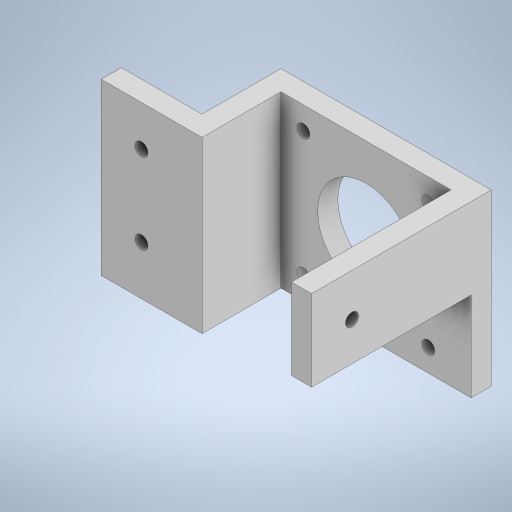
# Autodesk Inventor part: Motor Mount
Saved by Autodesk Inventor 2023.1 (Build 271208000, 208)
## iProperties
Created: 2022-10-30
Part Number: Motor Mount
Material: Generic
Document SubType Name: Modeling
Designer: nicol
Density: 1 g/cm^3
Appearance: Default
Author: nicol
Autodesk Inventor part; units mm, degrees
ref_plane "YZ Plane" through (0, 0, 0) normal (1, 0, 0) x (0, 1, 0)
ref_plane "XZ Plane" through (0, 0, 0) normal (0, 1, 0) x (-1, 0, 0)
ref_plane "XY Plane" through (0, 0, 0) normal (0, 0, 1) x (1, 0, 0)
sketch "Sketch1" plane through (0, 0, 0) normal (0, 0, 1) x (1, 0, 0)
  line L0 (0, 0) -> (42.2, 0)
  line L1 (42.2, 0) -> (42.2, 42.2)
  line L2 (42.2, 42.2) -> (0, 42.2)
  line L3 (0, 42.2) -> (0, 0)
  line L4 (0, 0) -> (5, 0)
  line L5 (42.2, 0) -> (45, 0)
  line L6 (5.6, 36.6) -> (36.6, 36.6) construction
  line L7 (36.6, 36.6) -> (36.6, 5.6) construction
  line L8 (36.6, 5.6) -> (5.6, 5.6) construction
  line L9 (5.6, 5.6) -> (5.6, 36.6) construction
  circle A0 centre (21.1, 21.1) radius 12
  line L10 (0.1, 42.1) -> (42.1, 42.1)
  line L11 (42.1, 42.1) -> (42.1, 0.1)
  line L12 (42.1, 0.1) -> (0.1, 0.1)
  line L13 (0.1, 0.1) -> (0.1, 42.1)
  line L14 (42.2, 42.2) -> (47.2, 42.2)
  line L15 (47.2, 42.2) -> (47.2, 21.1)
  line L16 (47.2, 21.1) -> (42.2, 21.1)
  line L17 (42.2, 21.1) -> (42.2, 42.2)
  line L18 (0, 42.2) -> (-5, 42.2)
  line L19 (-5, 42.2) -> (-5, 0)
  line L20 (-5, 0) -> (0, 0)
  line L21 (0, 0) -> (0, 42.2)
  point P0 (36.6, 21.1)
  point P1 (42.1, 21.1)
  point P2 (21.1, 36.6)
  point P3 (21.1, 42.1)
  point P4 (21.1, 42.2)
  dimension "d0" = 31
  dimension "d1" = 42
  dimension "d5" = 0.1
  dimension "d6" = 0.1
  dimension "d7" = 24
  dimension "d32" = 5
  dimension "d37" = 5
  constraints: 44 end point, 10 parallel, 8 perpendicular, 7 horizontal, 6 midpoint, 4 coincident, 3 vertical alignment, 2 horizontal alignment, 1 centre point, 1 collinear
  measures "d0" distance of L7.end L8.end
  measures "d1" distance of L10.end L11.end
  measures "d5" distance between parallel lines of L0 L12
  measures "d6" distance between parallel lines of L2 L10
  measures "d7" diameter of A0
  measures "d32" distance of L15.end L16.end
  measures "d37" distance of L2.end L18.end
extrude "Extrusion2" add sketch "Sketch1" along normal blind 5 contours L3 L2 L1 L0 | L10 L11 L12 L13
extrude "Extrusion4" add sketch "Sketch1" along normal blind 44.6 contours L14 L15 L16 L1
extrude "Extrusion5" add sketch "Sketch1" along normal blind 24.6 contours L20 L19 L18 L3
hole "Hole1" at (5.6, 36.6, 0) at (36.6, 36.6, 0) at (36.6, 5.6, 0) at (5.6, 5.6, 0) direction (0, 0, 1) diameter 3.2 end through all
sketch "Sketch4" plane through (42.2, 42.2, 44.6) normal (0, 1, 0) x (1, 0, 0)
  line L0 (-47.2, 20) -> (-67.2, 20)
  line L1 (-67.2, 20) -> (-67.2, 25)
  line L2 (-67.2, 25) -> (-47.2, 25)
  line L3 (-47.2, 25) -> (-47.2, 20)
  point P0 (-42.2, 44.6)
  dimension "d42" = 20
  dimension "d43" = 5
  constraints: 8 end point, 2 parallel, 1 horizontal, 1 perpendicular
  measures "d42" distance of L1.end L2.end
  measures "d43" distance of L0.end L1.end
extrude "Extrusion6" add sketch "Sketch4" against normal up to surface (42.2 mm away)
sketch "Sketch5" plane through (47.2, 21.1, 44.6) normal (1, 0, 0) x (0, 0, -1)
  line L0 (0, 0) -> (0, 21.1) projected
  line L1 (44.6, 21.1) -> (0, 21.1) projected
  line L2 (44.6, 0) -> (0, 0) projected
  point P0 (44.6, -21.1)
  point P1 (10, 10.55)
  point P2 (49.6, 26)
  point P3 (49.6, 0)
  dimension "d46" = 10
  dimension "d47" = 10.55
  dimension "d48" = 10.55
  constraints: 1 other
  measures "d46" distance from line of L0 point (10, 10.55)
  measures "d48" distance from line of L2 point (10, 10.55)
sketch "Sketch6" plane through (-5, 42.2, 19.6) normal (0, 0, -1) x (-1, 0, 0)
  line L0 (0, -42.2) -> (20, -42.2) projected
  line L1 (20, 0) -> (20, -42.2) projected
  line L2 (0, 0) -> (20, 0) projected
  line L3 (0, -42.2) -> (0, 0) projected
  point P0 (-5, -42.2)
  point P1 (10, -10)
  point P2 (10, -30)
  point P3 (10, -42.2)
  point P4 (10, 0)
  dimension "d49" = 10
  dimension "d65" = 20
  constraints: 3 vertical alignment, 2 midpoint
  measures "d49" distance from line of L2 point (10, -10)
  measures "d65" distance of point (10, -10) point (10, -30)
hole "Hole3" at (-15, 32.2, 19.6) at (-15, 12.2, 19.6) direction (0, 0, 1) diameter 3.2 end through all
hole "Hole4" at (47.2, 31.65, 34.6) direction (-1, 0, 0) diameter 3.2 end through all
sketch "Sketch7" plane through (42.2, 0, 5) normal (1, 0, 0) x (0, 0, -1)
  line L0 (5, 21.1) -> (0, 21.1) projected
  line L1 (0, 0) -> (0, 21.1) projected
  line L2 (5, 0) -> (0, 0) projected
  line L3 (5, 0) -> (5, 21.1) projected
  point P0 (5, 0)
extrude "Extrusion7" add sketch "Sketch7" along normal blind 5
thicken "Thicken2" operation cut thickness 1 both sides no extend neighbours no toward (0, 1, 0) faces at (45.5333, 21.1, 18.2)
equation "\"d6\" = d5"
equation "\"d47\" = d48"
body "Solid1"
